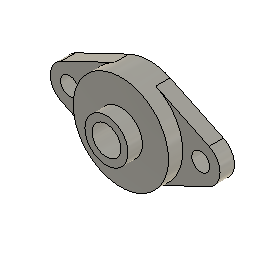
b89c69ff-4f11-40bf-9f73-3e73eaa56b80 (Autodesk Fusion 360 design; units mm, degrees)
Autodesk Fusion 360 part; units mm, degrees
sketch "Sketch1" plane through (0, 0, 0) normal (0, 1, 0) x (1, 0, 0)
  circle A0 centre (0, 0) radius 4
  line L0 (-18.25, 0) -> (18.25, 0)
  line L1 (18.25, 0) -> (18.25, 24.1955)
  line L2 (18.25, 24.1955) -> (-18.25, 24.1955)
  line L3 (-18.25, 24.1955) -> (-18.25, 0)
  circle A1 centre (-18.25, 0) radius 2.5
  circle A2 centre (18.25, 0) radius 2.5
  circle A3 centre (-18.25, 0) radius 5.375
  circle A4 centre (18.25, 0) radius 5.375
  line L4 (-23.625, 0) -> (23.625, 0)
  line L5 (23.625, 0) -> (23.625, -20.6716)
  line L6 (23.625, -20.6716) -> (-23.625, -20.6716)
  line L7 (-23.625, -20.6716) -> (-23.625, 0)
  circle A5 centre (0, 0) radius 13.25
  line L8 (-5.7175, -11.953) -> (-20.5693, -4.8488)
  line L9 (5.7175, -11.953) -> (20.5693, -4.8488)
  line L10 (5.7175, 11.953) -> (20.5693, 4.8488)
  line L11 (-5.7175, 11.953) -> (-20.5693, 4.8488)
  dimension "d1" = 8
  dimension "d2" = 5
  dimension "d3" = 5
  dimension "d4" = 18.25
  dimension "d5" = 18.25
  dimension "d6" = 10.75
  dimension "d7" = 10.75
  dimension "d8" = 45.5
  dimension "d9" = 26.5
  measures "d1" diameter of A0
  measures "d2" diameter of A1
  measures "d3" diameter of A2
  measures "d4" distance of A0.centre
  measures "d5" distance of A0.centre
  measures "d6" diameter of A3
  measures "d7" diameter of A4
  measures "d9" diameter of A5
extrude "Extrude1" add sketch "Sketch1" along normal blind 4 contours A0 L0 A3 A4 L4 A5 | A0 L0 A3 A4 L4 A5 | L0 A4 L4 A5 | L0 A4 L4 A5 | L0 A3 L4 A5 | L0 A3 L4 A5 | L0 L1 A2 A4 L4 A5 | L0 A2 A4 L4 A5 | L1 A4 A5 L10 | A4 A5 L9 | L0 A1 A3 L4 A5 | L0 L3 A1 A3 L4 A5 | L3 A3 A5 L11 | A3 A5 L8 | L1 A2 A4 L4 | L1 A4 L10 | L3 A3 L11 | L3 A1 A3 L4
sketch "Sketch2" plane through (0, 0, 0) normal (0, -1, 0) x (1, 0, 0)
  circle A0 centre (18.25, 0) radius 2.5
  circle A1 centre (0, 0) radius 4
  circle A2 centre (-18.25, 0) radius 2.5
  arc A3 (-5.7175, -11.953) -> (5.7175, -11.953) centre (0, 0) ccw
  line L0 (5.7175, -11.953) -> (20.5693, -4.8488)
  arc A4 (20.5693, -4.8488) -> (20.5693, 4.8488) centre (18.25, 0) ccw
  line L1 (20.5693, 4.8488) -> (5.7175, 11.953)
  arc A5 (5.7175, 11.953) -> (-5.7175, 11.953) centre (0, 0) ccw
  line L2 (-5.7175, 11.953) -> (-20.5693, 4.8488)
  arc A6 (-20.5693, 4.8488) -> (-20.5693, -4.8488) centre (-18.25, 0) ccw
  line L3 (-20.5693, -4.8488) -> (-5.7175, -11.953)
  circle A7 centre (0, 0) radius 13.25
extrude "Extrude2" add sketch "Sketch2" along normal blind 4 contours A3 A5 A7
sketch "Sketch3" plane through (0, -4, 0) normal (0, -1, 0) x (1, 0, 0)
  circle A0 centre (0, 0) radius 4
  circle A1 centre (0, 0) radius 13.25
  circle A2 centre (0, 0) radius 6
  dimension "d14" = 12
  measures "d14" diameter of A2
extrude "Extrude3" add sketch "Sketch3" along normal blind 4 contours A2
equation "d3 = d2"
equation "d4 = ( 36.5 / 2 ) * 1 mm"
equation "d5 = d4"
equation "d7 = d6"
